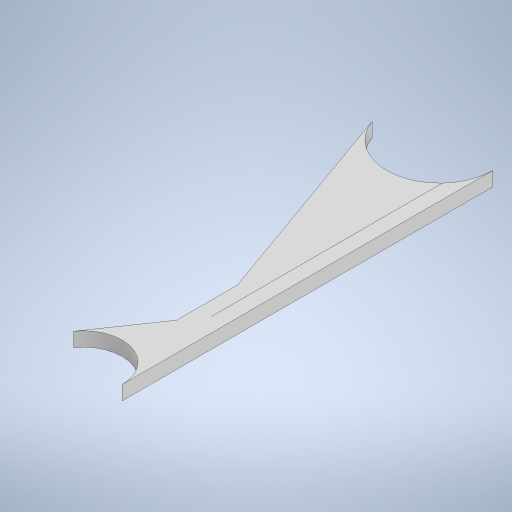
# Autodesk Inventor part: Podstavka
Saved by Autodesk Inventor 2024 (Build 280153000, 153)
## iProperties
Created: 2023-08-21
Part Number: Podstavka
Material: Generic
Document SubType Name: Modeling
Designer: KirikDK
Density: 1 g/cm^3
Appearance: Default
Author: KirikDK
Autodesk Inventor part; units mm, degrees
ref_plane "YZ Plane" through (0, 0, 0) normal (1, 0, 0) x (0, 1, 0)
ref_plane "XZ Plane" through (0, 0, 0) normal (0, 1, 0) x (-1, 0, 0)
ref_plane "XY Plane" through (0, 0, 0) normal (0, 0, 1) x (1, 0, 0)
sketch "Sketch1" plane through (0, 0, 0) normal (0, 1, 0) x (-1, 0, 0)
  line L0 (80.3147, 135.7125) -> (-79.6853, 135.7125)
  line L1 (-79.6853, 135.7125) -> (-79.6853, -314.2875)
  line L2 (-79.6853, -314.2875) -> (80.3147, -314.2875)
  line L3 (80.3147, -314.2875) -> (80.3147, 135.7125)
  line L4 (80.3147, 135.7125) -> (-79.7098, 135.7125)
  line L5 (-79.7098, 135.7125) -> (-79.7098, 335.7125)
  line L6 (-79.7098, 335.7125) -> (80.3147, 335.7125)
  line L7 (80.3147, 335.7125) -> (80.3147, 135.7125)
  line L8 (-79.7098, 135.7125) -> (80.3147, -314.2875)
  line L9 (-79.7098, 135.7125) -> (57.3679, 335.7125)
  line L10 (-79.7098, 335.7125) -> (-59.6853, 335.7125)
  line L11 (-59.6853, 335.7125) -> (-59.6853, -314.2875)
  line L12 (-59.6853, -314.2875) -> (-79.7098, -314.2875)
  line L13 (-79.7098, -314.2875) -> (-79.7098, 335.7125)
  line L14 (-79.7098, 335.7125) -> (-99.7098, 335.7125)
  line L15 (-99.7098, 335.7125) -> (-99.7098, -314.2875)
  line L16 (-99.7098, -314.2875) -> (-79.7098, -314.2875)
  line L17 (-79.7098, -314.2875) -> (-79.7098, 335.7125)
  circle A0 centre (-45.5025, 281.5053) radius 54.2073
  circle A1 centre (-25.2259, -239.8036) radius 74.4839
  point P0 (0, 0)
  point P1 (-5.6853, -93.2875)
  point P2 (44.9528, -214.8473)
  point P3 (-59.6853, 79.4024)
  point P4 (-59.6853, 164.9287)
  point P5 (-0.7894, 250.8594)
  point P6 (-99.7098, 281.5053)
  point P7 (-99.7098, -239.8036)
  point P8 (-79.7098, -189.0162)
  point P9 (-79.6853, -188.99)
  dimension "d0" = 450
  dimension "d1" = 200
  dimension "d2" = 160
  dimension "d3" = 20
  dimension "d4" = 20
  constraints: 36 end point, 8 parallel, 6 tangent, 4 horizontal, 4 perpendicular, 2 centre point, 2 point on line
  measures "d0" distance of L2.end L0.start
  measures "d1" distance of L6.end L0.start
  measures "d2" distance of L0.start L0.end
  measures "d3" distance between parallel lines of L1 L11
  measures "d4" distance between parallel lines of L13 L15
extrude "Extrusion1" add sketch "Sketch1" along normal blind 20 contours L11 L8 L1 L0 | L0 L4 L9 L11 | L11 A0 L9 | L9 L5 A0 L11 | L11 A1 L1 L8 | L8 A1 L11 | L13 A1 L15 A0 L5
body "Solid1"
